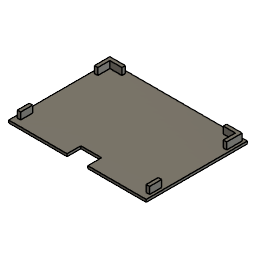
OTIS top panel (Autodesk Fusion 360 design; units mm, degrees)
part number: 2026-08-06-09-41-14-601
Autodesk Fusion 360 part; units mm, degrees
sketch "Sketch1" plane through (0, 0, 0) normal (0, 1, 0) x (1, 0, 0)
  line L0 (0, 0) -> (80, 0)
  line L1 (80, 0) -> (80, 58.89)
  line L2 (80, 58.89) -> (0, 58.89)
  line L3 (0, 58.89) -> (0, 0)
  line L4 (46, 0) -> (34, 0)
  line L5 (34, 0) -> (34, 8)
  line L6 (34, 8) -> (46, 8)
  line L7 (46, 8) -> (46, 0)
  dimension "d1" = 58.89
  dimension "d2" = 80
  dimension "d11" = 8
  dimension "d14" = 12
  dimension "d15" = 34
  constraint horizontal L0
  constraint vertical L1
  constraint horizontal L2
  constraint vertical L3
  constraint coincident L0.start L3.end
  constraint horizontal L4
  constraint vertical L5
  constraint horizontal L6
  constraint vertical L7
  constraint coincident L0 L4.start
  measures "d1" distance of L0.start L2.end
  measures "d2" distance of L1 L3
  measures "d11" distance of L4.end L5.end
  measures "d14" distance of L5.end L6.end
  measures "d15" distance of L3 L5
extrude "Extrude1" add sketch "Sketch1" along normal blind 1.5
sketch "Sketch2" plane through (0, 1.5, 0) normal (0, 1, 0) x (-1, 0, 0)
  line L0 (0, -58.89) -> (0, 0)
  line L1 (0, 0) -> (-80, 0)
  line L2 (-80, 0) -> (-80, -58.89)
  line L3 (-80, -58.89) -> (0, -58.89)
  line L4 (-10.51, -1.51) -> (-1.51, -1.51)
  line L5 (-1.51, -1.51) -> (-1.51, -10.51)
  line L6 (-1.51, -10.51) -> (-10.51, -10.51)
  line L7 (-10.51, -10.51) -> (-10.51, -1.51)
  line L8 (-10.51, -10.51) -> (-3.51, -10.51)
  line L9 (-3.51, -10.51) -> (-3.51, -3.51)
  line L10 (-3.51, -3.51) -> (-10.51, -3.51)
  line L11 (-10.51, -3.51) -> (-10.51, -10.51)
  line L12 (0, -29.445) -> (-80, -29.445) construction
  line L13 (-3.51, -48.38) -> (-3.51, -55.38)
  line L14 (-3.51, -55.38) -> (-10.51, -55.38)
  line L15 (-10.51, -48.38) -> (-10.51, -57.38)
  line L16 (-1.51, -48.38) -> (-10.51, -48.38)
  line L17 (-1.51, -57.38) -> (-1.51, -48.38)
  line L18 (-10.51, -57.38) -> (-1.51, -57.38)
  line L19 (-69.49, -1.51) -> (-78.49, -1.51)
  line L20 (-76.49, -3.51) -> (-69.49, -3.51)
  line L21 (-78.49, -1.51) -> (-78.49, -10.51)
  line L22 (-76.49, -10.51) -> (-76.49, -3.51)
  line L23 (-78.49, -10.51) -> (-69.49, -10.51)
  line L24 (-69.49, -10.51) -> (-69.49, -1.51)
  line L25 (-78.49, -48.38) -> (-69.49, -48.38)
  line L26 (-69.49, -48.38) -> (-69.49, -57.38)
  line L27 (-76.49, -48.38) -> (-76.49, -55.38)
  line L28 (-78.49, -57.38) -> (-78.49, -48.38)
  line L29 (-76.49, -55.38) -> (-69.49, -55.38)
  line L30 (-69.49, -57.38) -> (-78.49, -57.38)
  line L31 (-3.51, -3.51) -> (-1.51, -3.51)
  line L32 (-76.49, -3.51) -> (-78.49, -3.51)
  dimension "d5" = 9
  dimension "d6" = 9
  dimension "d7" = 1.51
  dimension "d8" = 1.51
  constraint horizontal L4
  constraint vertical L5
  constraint horizontal L6
  constraint vertical L7
  constraint horizontal L8
  constraint vertical L9
  constraint horizontal L10
  constraint vertical L11
  constraint coincident L5 L31.end
  constraint perpendicular L9 L31
  constraint coincident L21 L32.end
  constraint perpendicular L21 L32
  measures "d5" distance of L4.start L4.end
  measures "d6" distance of L4.start L6.end
  measures "d7" distance of L0 L5
  measures "d8" distance of L1 L4
extrude "Extrude2" add sketch "Sketch2" along normal blind 4 contours L5 L6 L9 L31 | L13 L14 L15 L16 L17 L18 | L21 L22 L23 L32 | L25 L26 L27 L28 L29 L30
extrude "Extrude3" cut sketch "Sketch1" along normal blind 8.263 contours L0 L4 L5 L6 L7
